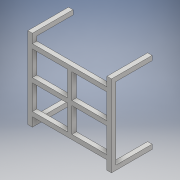
# Autodesk Inventor part: Raket_Holder
Saved by Autodesk Inventor 2018 (Build 220112000, 112)
## iProperties
Created: 2017-08-14
Part Number: Raket_Holder
Material: Generic
Document SubType Name: Modeling
Designer: andre
Density: 1 g/cm^3
Appearance: Default
Author: andre
## iProperties of the stored document Raket_Holder_3DPrint.ipt
Created: 2017-08-14
Part Number: Raket_Holder_3DPrint
Material: Generic
Document SubType Name: Modeling
Designer: andre
Density: 1 g/cm^3
Appearance: Default
Author: andre
Autodesk Inventor part; units mm, degrees
ref_plane "YZ Plane" through (0, 0, 0) normal (1, 0, 0) x (0, 1, 0)
ref_plane "XZ Plane" through (0, 0, 0) normal (0, 1, 0) x (-1, 0, 0)
ref_plane "XY Plane" through (0, 0, 0) normal (0, 0, 1) x (1, 0, 0)
sketch "Sketch1" plane through (0, 0, 0) normal (0, 1, 0) x (-1, 0, 0)
  line L0 (0, 0) -> (185, 0)
  line L1 (185, 0) -> (185, -140)
  line L2 (185, -140) -> (0, -140)
  line L3 (0, -140) -> (0, 0)
  line L4 (0, 0) -> (0, -10)
  line L5 (0, -10) -> (10, -10)
  line L6 (185, -140) -> (175, -140)
  line L7 (175, -140) -> (175, -130)
  line L8 (175, -130) -> (10, -130)
  line L9 (10, -130) -> (10, -10)
  line L10 (10, -10) -> (175, -10)
  line L11 (175, -10) -> (175, -130)
  line L12 (92.5, -130) -> (97.5, -130)
  line L13 (97.5, -130) -> (87.5, -130)
  line L14 (87.5, -130) -> (87.5, -10)
  line L15 (87.5, -10) -> (97.5, -10)
  line L16 (97.5, -10) -> (97.5, -130)
  line L17 (175, -70) -> (175, -75)
  line L18 (175, -75) -> (10, -75)
  line L19 (10, -75) -> (10, -65)
  line L20 (10, -65) -> (175, -65)
  line L21 (175, -65) -> (175, -75)
  dimension "d0" = 185
  dimension "d1" = 140
  dimension "d2" = 10
  dimension "d3" = 10
  dimension "d4" = 10
  dimension "d5" = 10
  dimension "d6" = 5
  dimension "d7" = 10
  dimension "d8" = 5
  dimension "d9" = 10
  constraints: 44 end point, 8 parallel, 6 perpendicular, 6 point on line, 4 horizontal, 2 midpoint
  measures "d0" distance of L1.end L2.end
  measures "d1" distance of L0.end L1.end
  measures "d2" distance of L0.start L4.end
  measures "d3" distance of L4.end L5.end
  measures "d4" distance of L1.end L6.end
  measures "d5" distance of L6.end L7.end
  measures "d6" distance of L12.start L12.end
  measures "d7" distance of L14.end L15.end
  measures "d8" distance of L17.start L17.end
  measures "d9" distance of L18.end L19.end
extrude "Extrusion1" add sketch "Sketch1" along normal blind 10 contours L0 L1 L2 L7 L11 L10 L5 L3 | L5 L9 L8 L7 L2 L3 | L20 L14 L18 L9 | L10 L16 L20 L14 | L20 L16 L18 L14 | L8 L14 L18 L16 | L18 L16 L20 L11
sketch "Sketch2" plane through (0, 0, -140) normal (0, 0, -1) x (-1, 0, 0)
  line L0 (185, 0) -> (0, 0) projected
  line L1 (175, 0) -> (175, 10) projected
  line L2 (185, 0) -> (175, 0)
  line L3 (175, 0) -> (175, 10)
  line L4 (175, 10) -> (185, 10)
  line L5 (185, 10) -> (185, 0)
  line L6 (10, 0) -> (10, 10) projected
  line L7 (0, 0) -> (10, 0)
  line L8 (10, 0) -> (10, 10)
  line L9 (10, 10) -> (0, 10)
  line L10 (0, 10) -> (0, 0)
  dimension "d12" = 10
  dimension "d13" = 10
  dimension "d14" = 10
  constraints: 16 end point, 4 parallel, 2 horizontal, 2 perpendicular
  measures "d12" distance of L1.end L4.end
  measures "d13" distance of L9.end L6.end
  measures "d14" distance of L6.end L7.end
extrude "Extrusion2" add sketch "Sketch2" along normal blind 20
sketch "Sketch3" plane through (-185, 0, 0) normal (0, 0, 1) x (1, 0, 0)
  line L0 (0, 10) -> (10, 10) projected
  line L1 (87.5, 0) -> (10, 0) projected
  line L2 (0, 10) -> (10, 10)
  line L3 (10, 10) -> (10, 0)
  line L4 (10, 0) -> (0, 0)
  line L5 (0, 0) -> (0, 10)
  line L6 (185, 0) -> (185, 10) projected
  line L7 (175, 0) -> (97.5, 0) projected
  line L8 (185, 10) -> (175, 10)
  line L9 (175, 10) -> (175, 0)
  line L10 (175, 0) -> (185, 0)
  line L11 (185, 0) -> (185, 10)
  dimension "d17" = 10
  constraints: 16 end point, 4 parallel, 2 horizontal, 2 perpendicular
  measures "d17" distance of L10.end L7.start
extrude "Extrusion3" add sketch "Sketch3" along normal blind 20
sketch "Sketch4" plane through (0, 10, 0) normal (0, 1, 0) x (1, 0, 0)
  line L0 (-185, -20) -> (-185, 160) projected
  line L1 (-175, 0) -> (-175, -20) projected
  line L2 (-185, -20) -> (-175, -20)
  line L3 (-175, -20) -> (-175, -10)
  line L4 (-175, -10) -> (-185, -10)
  line L5 (-185, -10) -> (-185, -20)
  line L6 (-175, 140) -> (-175, 160) projected
  line L7 (-185, 160) -> (-175, 160)
  line L8 (-175, 160) -> (-175, 150)
  line L9 (-175, 150) -> (-185, 150)
  line L10 (-185, 150) -> (-185, 160)
  line L11 (-10, 160) -> (0, 160) projected
  line L12 (0, 160) -> (0, -20) projected
  line L13 (-10, 160) -> (0, 160)
  line L14 (0, 160) -> (0, 150)
  line L15 (0, 150) -> (-10, 150)
  line L16 (-10, 150) -> (-10, 160)
  line L17 (-10, -20) -> (0, -20) projected
  line L18 (-10, 0) -> (-10, -20) projected
  line L19 (0, -20) -> (-10, -20)
  line L20 (-10, -20) -> (-10, -15)
  line L21 (0, -15) -> (0, -20)
  line L22 (0, -20) -> (0, 160) projected
  line L23 (-10, 0) -> (-10, -20) projected
  line L24 (0, -20) -> (-10, -20)
  line L25 (-10, -20) -> (-10, -10)
  line L26 (-10, -10) -> (0, -10)
  line L27 (0, -10) -> (0, -20)
  point P0 (0, 0)
  dimension "d20" = 10
  dimension "d21" = 10
  dimension "d22" = 10
  dimension "d50" = 10
  constraints: 38 end point, 9 parallel, 5 horizontal, 5 perpendicular, 3 midpoint, 2 point on line
  measures "d20" distance of L3.end L2.end
  measures "d21" distance of L7.end L8.end
  measures "d22" distance of L13.end L14.end
  measures "d50" distance of L24.end L25.end
extrude "Extrusion4" add sketch "Sketch4" along normal blind 80
sketch "Sketch7" plane through (0, 90, 0) normal (0, 1, 0) x (1, 0, 0)
  line L0 (-10, -20) -> (0, -20) projected
  line L1 (-5, -20) -> (-5, -15)
  line L2 (0, 160) -> (-10, 160) projected
  line L3 (-5, 160) -> (-5, 155)
  circle A0 centre (-5, 155) radius 2.4
  circle A1 centre (-5, -15) radius 2.4
  circle A2 centre (-180, -15) radius 2.4
  circle A3 centre (-180, 155) radius 2.4
  point P0 (0, 0)
  dimension "d40" = 5
  dimension "d41" = 5
  dimension "d42" = 4.8
  dimension "d47" = 4.8
  dimension "d48" = 4.8
  dimension "d49" = 4.8
  constraints: 4 centre point, 4 end point, 2 coincident, 2 midpoint, 2 vertical
  measures "d40" distance of L1.start L1.end
  measures "d41" distance of L3.start L3.end
  measures "d42" diameter of A0
  measures "d47" diameter of A1
  measures "d48" diameter of A2
  measures "d49" diameter of A3
extrude "Extrusion7" cut sketch "Sketch7" against normal blind 25
body "Solid1"
